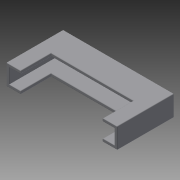
# Autodesk Inventor part: PhoneHolder
Saved by Autodesk Inventor 2015 (Build 190159000, 159)
## iProperties
Created: 2015-11-10
Part Number: PhoneHolder
Material: Generic
Document SubType Name: Modeling
Designer: Lauszus
Density: 1 g/cm^3
Appearance: Default
Author: Lauszus
Autodesk Inventor part; units mm, degrees
ref_plane "YZ Plane" through (0, 0, 0) normal (1, 0, 0) x (0, 1, 0)
ref_plane "XZ Plane" through (0, 0, 0) normal (0, 1, 0) x (-1, 0, 0)
ref_plane "XY Plane" through (0, 0, 0) normal (0, 0, 1) x (1, 0, 0)
sketch "Sketch1" plane through (0, 0, 0) normal (0, 1, 0) x (-1, 0, 0)
  line L0 (58.6433, 33) -> (-10.1567, 33)
  line L1 (-10.1567, 33) -> (-10.1567, 0)
  line L2 (-10.1567, 0) -> (58.6433, 0)
  line L3 (58.6433, 0) -> (58.6433, 33)
  line L4 (51.1433, 33) -> (51.1433, 15)
  line L5 (51.1433, 15) -> (-2.6567, 15)
  line L6 (-2.6567, 15) -> (-2.6567, 33)
  point P0 (0, 0)
  dimension "d12" = 68.8
  dimension "d13" = 33
  dimension "d14" = 7.5
  dimension "d15" = 7.5
  dimension "d16" = 15
  constraints: 14 end point, 3 perpendicular, 2 parallel, 2 point on line, 1 horizontal, 1 vertical
  measures "d12" distance of L1.end L2.end
  measures "d13" distance of L2.end L0.start
  measures "d14" distance between parallel lines of L3 L4
  measures "d15" distance between parallel lines of L1 L6
  measures "d16" distance between parallel lines of L2 L5
extrude "Extrusion1" add sketch "Sketch1" along normal blind 9.5 contours L3 L2 L1 L0 L6 L5 L4
shell "Shell1" thickness 2 outward yes removed faces 3 at (-33.21, 3.1667, 15) at (-51.1433, 3.1667, 27) at (2.6567, 3.1667, 21)
sketch "Sketch7" plane through (-58.6433, 0, 0) normal (0, 0, 1) x (1, 0, 0)
  line L0 (68.8, 0) -> (68.8, 9.5) projected
  line L1 (68.8, 4.75) -> (0, 4.75)
  line L2 (0, 0) -> (0, 9.5) projected
  circle A0 centre (17.2, 4.75) radius 1
  line L3 (34.4, 10) -> (34.4, 0)
  circle A1 centre (51.6, 4.75) radius 1
  line L4 (70.8, -2) -> (70.8, 11.5) projected
  point P0 (58.6433, 0)
  dimension "d26" = 2
  dimension "d41" = 17.2
  dimension "d43" = 34.4
  constraints: 4 end point, 2 centre point, 2 midpoint, 1 point on line, 1 symmetric about line, 1 vertical, 1 other
  measures "d26" diameter of A0
  measures "d41" distance from line of A1.centre L3
  measures "d43" distance between parallel lines of L0 L3
hole "Hole1" at (-41.4433, 4.75, 0) at (-7.0433, 4.75, 0) direction (0, 0, -1) diameter 2 end through all countersink diameter 6 countersink angle 90
sketch "Sketch8" plane through (12.1567, -2, -2) normal (0, 0, -1) x (-1, 0, 0)
  line L0 (30.4, 9.75) -> (42.4, 9.75)
  line L1 (42.4, 9.75) -> (42.4, 3.75)
  line L2 (42.4, 3.75) -> (30.4, 3.75)
  line L3 (30.4, 3.75) -> (30.4, 9.75)
  line L4 (0, 0) -> (0, 13.5) projected
  line L5 (0, 13.5) -> (72.8, 13.5) projected
  point P0 (12.1567, 2)
  dimension "d35" = 12
  dimension "d36" = 6
  dimension "d37" = 30.4
  dimension "d38" = 3.75
  constraints: 8 end point, 2 parallel, 1 horizontal, 1 perpendicular
  measures "d35" distance of L1.end L2.end
  measures "d36" distance of L0.end L1.end
  measures "d37" distance between parallel lines of L4 L3
  measures "d38" distance between parallel lines of L5 L0
extrude "Extrusion6" cut sketch "Sketch8" against normal up to next
sketch "Sketch9" plane through (-60.6433, -2, 35) normal (0, 0, 1) x (1, 0, 0)
  line L0 (9.5, 0) -> (9.5, 13.5) projected
  line L1 (2, 2) -> (9.5, 2)
  line L2 (9.5, 2) -> (9.5, 11.5)
  line L3 (9.5, 11.5) -> (2, 11.5)
  line L4 (2, 11.5) -> (2, 2)
  line L5 (63.3, 11.5) -> (70.8, 11.5)
  line L6 (70.8, 11.5) -> (70.8, 2)
  line L7 (70.8, 2) -> (63.3, 2)
  line L8 (63.3, 2) -> (63.3, 11.5)
  point P0 (60.6433, 2)
  constraints: 16 end point, 4 parallel, 2 horizontal, 2 perpendicular, 1 point on line
extrude "Extrusion7" cut sketch "Sketch9" against normal up to next
fillet "Fillet1" radius 0.4 28 edges at (-54.8933, 9.5, 35) (-58.6433, 4.75, 35) (-54.8933, 0, 35) (6.4067, 0, 35) (10.1567, 4.75, 35) (6.4067, 9.5, 35) (-55.8933, 11.5, 35) (-60.6433, 4.75, 35) (-55.8933, -2, 35) (-60.6433, -2, 16.5) (-60.6433, 11.5, 16.5) (2.6567, 9.5, 25) (2.6567, 11.5, 25) (-24.2433, 11.5, 15) (-24.2433, 9.5, 15) (2.6567, -2, 25) (2.6567, 0, 25) (-24.2433, 0, 15) (-24.2433, -2, 15) (7.4067, -2, 35) (12.1567, 4.75, 35) (7.4067, 11.5, 35) (-51.1433, 9.5, 25) (-51.1433, 0, 25) (12.1567, 11.5, 16.5) (12.1567, -2, 16.5) (-51.1433, -2, 25) (-51.1433, 11.5, 25)
body "Solid2"
